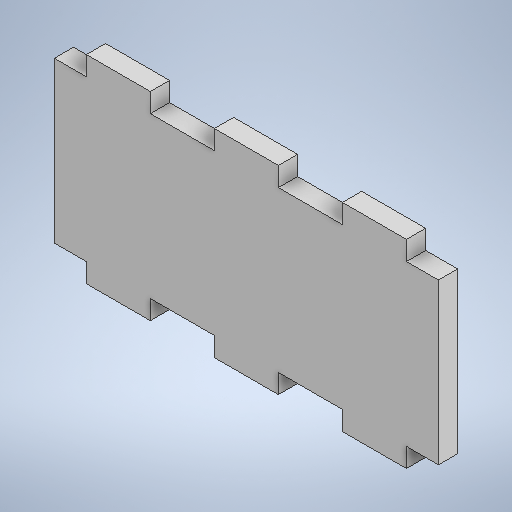
# Autodesk Inventor part: Base Connection
Saved by Autodesk Inventor 2025.3 (Build 293356000, 356)
## iProperties
Created: 2026-04-16
Part Number: Base Connection
Material: Generic
Document SubType Name: Modeling
Designer: ziada
Density: 1 g/cm^3
Appearance: Default
Author: ziada
Autodesk Inventor part; units mm, degrees
ref_plane "YZ Plane" through (0, 0, 0) normal (1, 0, 0) x (0, 1, 0)
ref_plane "XZ Plane" through (0, 0, 0) normal (0, 1, 0) x (-1, 0, 0)
ref_plane "XY Plane" through (0, 0, 0) normal (0, 0, 1) x (1, 0, 0)
sketch "Sketch1" plane through (0, 0, 0) normal (0, 0, 1) x (1, 0, 0)
  line L0 (0, 0) -> (0, 6)
  line L1 (0, 6) -> (10, 6)
  line L2 (10, 6) -> (10, 0)
  line L3 (10, 0) -> (30, 0)
  line L4 (30, 0) -> (30, 6)
  line L5 (30, 6) -> (50, 6)
  line L6 (50, 6) -> (50, 0)
  line L7 (50, 0) -> (70, 0)
  line L8 (70, 0) -> (70, 6)
  line L9 (70, 6) -> (90, 6)
  line L10 (90, 6) -> (90, 0)
  line L11 (90, 0) -> (110, 0)
  line L12 (110, 0) -> (110, 6)
  line L13 (110, 6) -> (120, 6)
  line L14 (120, 6) -> (120, 1)
  line L15 (0, 56) -> (10, 56)
  line L16 (10, 56) -> (10, 62)
  line L17 (10, 62) -> (30, 62)
  line L18 (30, 62) -> (30, 56)
  line L19 (30, 56) -> (50, 56)
  line L20 (50, 56) -> (50, 62)
  line L21 (50, 62) -> (70, 62)
  line L22 (70, 62) -> (70, 56)
  line L23 (70, 56) -> (90, 56)
  line L24 (90, 56) -> (90, 62)
  line L25 (90, 62) -> (110, 62)
  line L26 (110, 62) -> (110, 56)
  line L27 (110, 56) -> (120, 56)
  line L28 (0, 56) -> (0, 6)
  line L29 (120, 56) -> (120, 6)
  dimension "d0" = 6
  dimension "d1" = 10
  dimension "d2" = 20
  dimension "d3" = 20
  dimension "d4" = 20
  dimension "d5" = 20
  dimension "d6" = 20
  dimension "d8" = 10
  dimension "d12" = 10
  dimension "d13" = 6
  dimension "d14" = 20
  dimension "d15" = 50
  constraints: 60 end point, 18 perpendicular, 16 point on line, 3 parallel, 2 horizontal, 2 vertical
  measures "d0" distance of L0.start L0.end
  measures "d1" distance of L0.end L1.end
  measures "d2" distance of L2.end L3.end
  measures "d3" distance of L4.end L5.end
  measures "d4" distance of L6.end L7.end
  measures "d5" distance of L8.end L9.end
  measures "d6" distance of L10.end L11.end
  measures "d8" distance of L12.end L13.end
  measures "d12" distance of L15.start L15.end
  measures "d13" distance of L15.end L16.end
  measures "d14" distance of L16.end L17.end
  measures "d15" distance of L27.end L13.end
extrude "Extrusion1" add sketch "Sketch1" against normal blind 6
body "Solid1"
